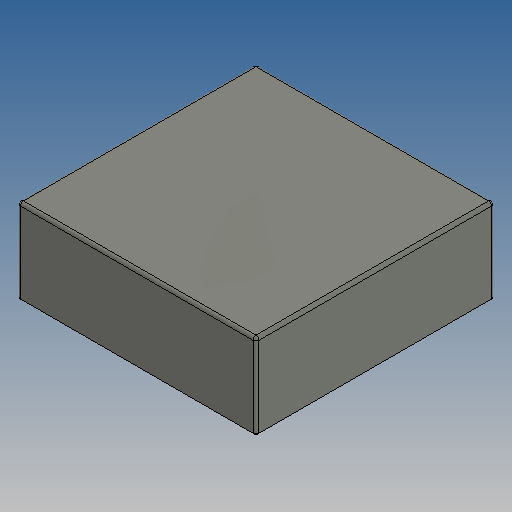
# Autodesk Inventor part: 3070b-DkBluishGray
Saved by Autodesk Inventor 2025 (Build 290162010, 162A)
## iProperties
Created: 2014-06-03
Part Number: 3070b-DkBluishGray
Material: ABS Plastic
Document SubType Name: Modeling
Designer: D. Kohfeld
Density: 1.06 g/cm^3
Appearance: DkBluishGray
Mass: 0.172759 g
Surface Area: 2.57972 cm^2
Volume: 0.16298 cm^3
Author: D. Kohfeld
Autodesk Inventor part; units mm, degrees
ref_plane "YZ Plane" through (0, 0, 0) normal (1, 0, 0) x (0, 1, 0)
ref_plane "XZ Plane" through (0, 0, 0) normal (0, 1, 0) x (-1, 0, 0)
ref_plane "XY Plane" through (0, 0, 0) normal (0, 0, 1) x (1, 0, 0)
sketch "Sketch2" plane through (0, 0, 0) normal (0, 1, 0) x (-1, 0, 0)
  line L0 (-4, 4) -> (4, 4)
  line L1 (4, 4) -> (4, -4)
  line L2 (4, -4) -> (-4, -4)
  line L3 (-4, -4) -> (-4, 4)
  point P0 (0, 0)
  point P1 (0, 4)
  point P2 (-4, 0)
  dimension "d0" = 8
  dimension "d1" = 8
  constraints: 8 end point, 2 midpoint, 2 parallel, 1 horizontal, 1 horizontal alignment, 1 perpendicular, 1 vertical alignment
  measures "d0" distance of L1.end L2.end
  measures "d1" distance of L2.end L0.start
extrude "Extrusion1" add sketch "Sketch2" along normal blind 3.2
sketch "Sketch3" plane through (0, 0, 0) normal (0, -1, 0) x (1, 0, 0)
  line L0 (4, 4) -> (-4, 4) projected
  line L1 (-4, 4) -> (-4, -4) projected
  line L2 (-2.4, 2.4) -> (2.4, 2.4)
  line L3 (2.4, 2.4) -> (2.4, -2.4)
  line L4 (2.4, -2.4) -> (-2.4, -2.4)
  line L5 (-2.4, -2.4) -> (-2.4, 2.4)
  line L6 (-4, -4) -> (4, -4) projected
  line L7 (4, -4) -> (4, 4) projected
  line L8 (-3.6, 3.6) -> (3.6, 3.6)
  line L9 (3.6, 3.6) -> (3.6, -3.6)
  line L10 (3.6, -3.6) -> (-3.6, -3.6)
  line L11 (-3.6, -3.6) -> (-3.6, 3.6)
  point P0 (0, 0)
  point P1 (-2.4, 0)
  point P2 (0, 2.4)
  point P3 (0, 0)
  point P4 (-3.6, 0)
  point P5 (0, 3.6)
  dimension "d8" = 1.6
  dimension "d62" = 1.6
  dimension "d98" = 0.4
  dimension "d99" = 0.4
  constraints: 16 end point, 4 midpoint, 4 parallel, 2 horizontal, 2 horizontal alignment, 2 perpendicular, 2 vertical alignment, 1 coincident
  measures "d8" distance between parallel lines of L1 L5
  measures "d62" distance between parallel lines of L0 L2
  measures "d98" distance between parallel lines of L0 L8
  measures "d99" distance between parallel lines of L1 L11
extrude "Extrusion2" cut sketch "Sketch3" against normal blind 1.6 contours L2 L3 L4 L5
extrude "Extrusion7" cut sketch "Sketch3" against normal blind 0.4 contours L7 L6 L1 L0
fillet "Fillet1" radius 0.1 8 edges at (-4, 1.8, 4) (0, 3.2, 4) (-4, 3.2, 0) (4, 1.8, 4) (4, 3.2, 0) (0, 3.2, -4) (4, 1.8, -4) (-4, 1.8, -4)
equation "\"d4\" = 0.333333 * lh"
equation "\"d8\" = d62"
equation "\"d62\" = wall"
equation "\"d98\" = gw"
equation "\"d99\" = d98"
equation "\"d11\" = 0.333333 * lh - topthk"
equation "\"d100\" = gh"
equation "\"d22\" = lf"
equation "\"lh\" = 9.6"
equation "\"wall\" = 1.6"
equation "\"gw\" = 0.4"
equation "\"topthk\" = 1.6"
equation "\"gh\" = 0.4"
equation "\"lf\" = 0.1"
body "Solid1"
